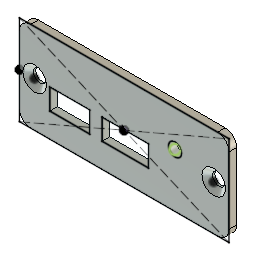
BMW-N57_Oilpress_Case (Autodesk Fusion 360 design; units mm, degrees)
Autodesk Fusion 360 part; units mm, degrees
note: some values were not read from the file. Set by a fixed rule: the direction of a hole.
sketch "Skizze1" plane through (0, 0, 0) normal (0, 1, 0) x (1, 0, 0)
  line L0 (27.5, 11.8) -> (-27.5, 11.8)
  line L1 (-27.5, 11.8) -> (-27.5, -11.8)
  line L2 (-27.5, -11.8) -> (27.5, -11.8)
  line L3 (27.5, -11.8) -> (27.5, 11.8)
  line L4 (27.5, 11.8) -> (-27.5, -11.8) construction
  line L5 (-27.5, 11.8) -> (27.5, -11.8) construction
  line L6 (-19.5, -0.1) -> (-9, -0.1)
  line L7 (-9, -0.1) -> (-9, 5.4)
  line L8 (-9, 5.4) -> (-19.5, 5.4)
  line L9 (-19.5, 5.4) -> (-19.5, -0.1)
  line L10 (-5.8, -0.1) -> (6.4, -0.1)
  line L11 (6.4, -0.1) -> (6.4, 5.4)
  line L12 (6.4, 5.4) -> (-5.8, 5.4)
  line L13 (-5.8, 5.4) -> (-5.8, -0.1)
  circle A0 centre (13.3661, -2.3066) radius 1.7
  point P0 (-27.5, 0)
  point P1 (-23.5, 0)
  point P2 (23.5, 0)
  dimension "d1" = 55
  dimension "d2" = 23.6
  dimension "d3" = 10.5
  dimension "d4" = 5.5
  dimension "d5" = 5.5
  dimension "d6" = 12.2
  dimension "d7" = 3.2
  dimension "d8" = 6.4
  dimension "d9" = 8
  dimension "d10" = 3.4
  dimension "d17" = 47
  dimension "d18" = 23.5
  constraint horizontal L0
  constraint perpendicular L0 L1
  constraint parallel L0 L2
  constraint parallel L1 L3
  constraint coincident L4 origin
  constraint coincident L5 origin
  constraint horizontal L6
  constraint vertical L7
  constraint horizontal L8
  constraint vertical L9
  constraint horizontal L10
  constraint vertical L11
  constraint horizontal L12
  constraint vertical L13
  constraint horizontal L8.end L12.end
  constraint midpoint L1 P0
  constraint horizontal P1 P2
  constraint horizontal P0 P1
  measures "d1" distance of L1.end L2.end
  measures "d2" distance of L0.end L1.end
  measures "d3" distance of L6.start L6.end
  measures "d4" distance of L6.start L8.end
  measures "d5" distance of L10.start L12.end
  measures "d6" distance of L10.start L10.end
  measures "d7" distance of L7 L13
  measures "d8" distance of L0 L8
  measures "d9" distance of L1 L9
  measures "d10" diameter of A0
  measures "d17" distance of P1 P2
  measures "d18" distance of origin P2
extrude "Extrusion1" add sketch "Skizze1" along normal blind 2
hole "Bohrung1" at (23.5, 0, 0) at (-23.5, 0, 0) direction (0, 1, 0) diameter 3.4 end through all countersink diameter 6.2 countersink angle 90
fillet "Abrundung1" radius 3 4 edges at (27.5, 1, 11.8) (-27.5, 1, 11.8) (-27.5, 1, -11.8) (27.5, 1, -11.8)
equation "d5 = d4"
equation "d18 = d17 / 2"
named bodies: "N57_Oilpress_Case_Deckel"
